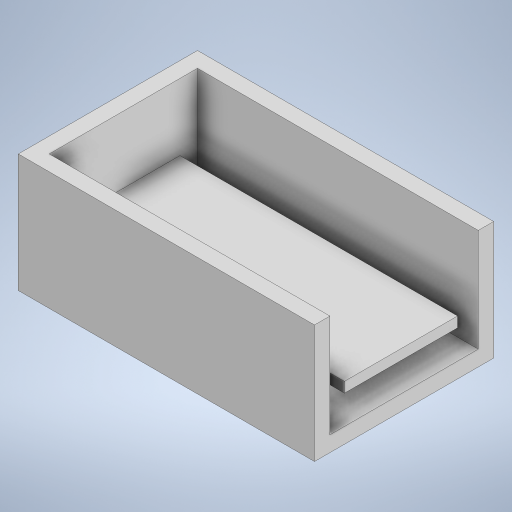
# Autodesk Inventor part: DudukanESP32
Saved by Autodesk Inventor 2024 (Build 280153000, 153)
## iProperties
Created: 2025-12-17
Part Number: DudukanESP32
Material: Generic
Document SubType Name: Modeling
Designer: risda
Density: 1 g/cm^3
Appearance: Default
Author: risda
Autodesk Inventor part; units mm, degrees
ref_plane "YZ Plane" through (0, 0, 0) normal (1, 0, 0) x (0, 1, 0)
ref_plane "XZ Plane" through (0, 0, 0) normal (0, 1, 0) x (-1, 0, 0)
ref_plane "XY Plane" through (0, 0, 0) normal (0, 0, 1) x (1, 0, 0)
sketch "Sketch1" plane through (0, 0, 0) normal (0, 1, 0) x (-1, 0, 0)
  line L0 (0, 0) -> (0, -28.85)
  line L1 (0, -28.85) -> (-51.6, -28.85)
  line L2 (0, 0) -> (-51.6, 0)
  line L3 (-51.6, 0) -> (-51.6, -28.85)
  line L4 (-54.6, -31.85) -> (3, -31.85)
  line L5 (3, -31.85) -> (3, 3)
  line L6 (3, 3) -> (-54.6, 3)
  line L7 (-54.6, 3) -> (-54.6, -31.85)
  dimension "d0" = 28.85
  dimension "d1" = 51.6
  dimension "d2" = 3
  constraints: 16 end point, 2 horizontal, 2 perpendicular, 1 vertical, 3 other
  measures "d0" distance of L0.start L0.end
  measures "d1" distance of L0.end L1.end
  measures "d2" distance between parallel lines of L1 L4
extrude "Extrusion1" add sketch "Sketch1" along normal blind 3 contours L0 L1 L3 L2
extrude "Extrusion2" add sketch "Sketch1" along normal blind 23
sketch "Sketch2" plane through (54.6, 0, 3) normal (1, 0, 0) x (0, 0, -1)
  line L0 (3, 3) -> (3, 23) projected
  line L1 (3, 23) -> (3, 3)
  line L2 (31.85, 3) -> (31.85, 23) projected
  line L3 (3, 3) -> (31.85, 3)
  line L4 (31.85, 3) -> (31.85, 23)
  line L5 (31.85, 23) -> (3, 23)
  point P0 (3, 0)
  constraints: 8 end point, 3 perpendicular, 1 vertical
extrude "Extrusion3" cut sketch "Sketch2" against normal blind 23
sketch "Sketch3" plane through (0, 3, -28.85) normal (1, 0, 0) x (0, 0, -1)
  line L0 (0, 0) -> (-28.85, 0) projected
  line L1 (-14.425, 0) -> (-14.425, 5)
  line L2 (-14.425, 5) -> (-3.425, 5)
  line L3 (-14.425, 5) -> (-25.425, 5)
  line L4 (-25.425, 5) -> (-25.425, 7)
  line L5 (-25.425, 7) -> (-3.425, 7)
  line L6 (-3.425, 7) -> (-3.425, 5)
  point P0 (-28.85, -3)
  dimension "d9" = 5
  dimension "d10" = 11
  dimension "d11" = 11
  dimension "d12" = 2
  constraints: 12 end point, 2 horizontal, 2 perpendicular, 2 vertical, 1 midpoint
  measures "d9" distance of L1.start L1.end
  measures "d10" distance of L1.end L2.end
  measures "d11" distance of L1.end L3.end
  measures "d12" distance of L3.end L4.end
extrude "Extrusion4" add sketch "Sketch3" along normal blind 54
body "Solid1"
